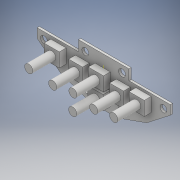
# Autodesk Inventor part: Keyboard1
Saved by Autodesk Inventor 2017 (Build 210142000, 142)
## iProperties
Created: 2017-04-18
Part Number: Keyboard1
Material: Generic
Document SubType Name: Modeling
Designer: Oleg
Density: 1 g/cm^3
Appearance: Default
Author: Oleg
Autodesk Inventor part; units mm, degrees
ref_plane "YZ Plane" through (0, 0, 0) normal (1, 0, 0) x (0, 1, 0)
ref_plane "XZ Plane" through (0, 0, 0) normal (0, 1, 0) x (-1, 0, 0)
ref_plane "XY Plane" through (0, 0, 0) normal (0, 0, 1) x (1, 0, 0)
sketch "Sketch1" plane through (0, 0, 0) normal (0, 1, 0) x (-1, 0, 0)
  circle A0 centre (48.634, 12.202) radius 1.778
  circle A1 centre (29.509, 5.597) radius 1.778
  circle A2 centre (37, 18) radius 1.5
  circle A3 centre (21, 18) radius 1.5
  circle A4 centre (3, 13.5) radius 1.5
  circle A5 centre (21, 4) radius 1.5
  circle A6 centre (37, 4) radius 1.5
  circle A7 centre (55, 13.5) radius 1.5
  circle A8 centre (11.639, 12.326) radius 1.778
  circle A9 centre (20.363, 11.115) radius 1.778
  circle A10 centre (29.407, 12.701) radius 1.778
  circle A11 centre (38.211, 11.232) radius 1.778
  line L0 (10.2856, 4.4998) -> (-0.0002, 12.5003)
  line L1 (34.6899, 0.0005) -> (47.7142, 4.5002)
  line L2 (57.9997, 16.5) -> (40.0003, 16.5)
  line L3 (39.9997, 21) -> (17.9997, 21)
  line L4 (-0.0003, 16.5) -> (18.0003, 16.5)
  line L5 (10.2856, 4.4998) -> (23.0001, 0.0002)
  line L6 (47.7142, 4.5002) -> (57.9998, 12.5002)
  line L7 (57.9997, 16.5) -> (57.9998, 12.5002)
  line L8 (34.6899, 0.0005) -> (23.0001, 0.0002)
  line L9 (-0.0002, 12.5003) -> (-0.0003, 16.5)
  line L10 (18.0003, 16.5) -> (17.9997, 21)
  line L11 (39.9997, 21) -> (40.0003, 16.5)
  line L12 (51.9741, 15.2119) -> (45.332, 15.2119)
  line L13 (45.332, 15.2119) -> (45.332, 9.1159)
  line L14 (45.332, 9.1159) -> (51.9741, 9.1159)
  line L15 (51.9741, 9.1159) -> (51.9741, 15.2119)
  line L16 (41.259, 14.534) -> (35.2011, 14.534)
  line L17 (35.2011, 14.534) -> (35.2011, 7.93)
  line L18 (35.2011, 7.93) -> (41.259, 7.93)
  line L19 (41.259, 7.93) -> (41.259, 14.534)
  line L20 (32.7471, 15.7871) -> (26.105, 15.7871)
  line L21 (26.105, 15.7871) -> (26.105, 9.6911)
  line L22 (26.105, 9.6911) -> (32.7471, 9.6911)
  line L23 (32.7471, 9.6911) -> (32.7471, 15.7871)
  line L24 (32.8491, 8.6831) -> (26.207, 8.6831)
  line L25 (26.207, 8.6831) -> (26.207, 2.549)
  line L26 (26.207, 2.549) -> (32.8491, 2.549)
  line L27 (32.8491, 2.549) -> (32.8491, 8.6831)
  line L28 (23.4491, 14.417) -> (17.3531, 14.417)
  line L29 (17.3531, 14.417) -> (17.3531, 7.7749)
  line L30 (17.3531, 7.7749) -> (23.4491, 7.7749)
  line L31 (23.4491, 7.7749) -> (23.4491, 14.417)
  line L32 (14.9791, 15.4121) -> (8.337, 15.4121)
  line L33 (8.337, 15.4121) -> (8.337, 9.337)
  line L34 (8.337, 9.337) -> (14.9791, 9.337)
  line L35 (14.9791, 9.337) -> (14.9791, 15.4121)
  point P0 (0, 0)
  constraints: 72 end point, 14 parallel, 12 centre point, 8 horizontal, 8 perpendicular, 46 other
extrude "Extrusion1" add sketch "Sketch1" along normal blind 1 contours A0 | A1 | A8 | A9 | A10 | A11 | L0 L9 L4 L10 L3 L11 L2 L7 L6 L1 L8 L5 | L15 L14 L13 L12 | L19 L18 L17 L16 | L23 L22 L21 L20 | L27 L26 L25 L24 | L31 L30 L29 L28 | L35 L34 L33 L32
extrude "Extrusion2" add sketch "Sketch1" against normal blind 3 contours L15 L14 L13 L12 | L19 L18 L17 L16 | L23 L22 L21 L20 | L27 L26 L25 L24 | L31 L30 L29 L28 | L35 L34 L33 L32
extrude "Extrusion3" add sketch "Sketch1" against normal blind 13 contours A0 | A1 | A8 | A9 | A10 | A11
ref_plane "Work Plane1" through (-28.9998, 0, 12.501) normal (1, 0, 0) x (0, 0, -1)
body "Solid1"
